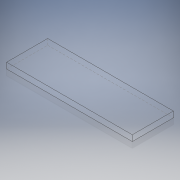
# Autodesk Inventor part: Door Shelf
Saved by Autodesk Inventor 2016 (Build 200138000, 138)
## iProperties
Created: 2017-10-31
Part Number: Door Shelf
Material: Wood (Cherry)
Document SubType Name: Modeling
Designer: mathaetaes
Density: 0.63 g/cm^3
Appearance: Cherry - Natural Low Gloss
Author: mathaetaes
Autodesk Inventor part; units mm, degrees
ref_plane "YZ Plane" through (0, 0, 0) normal (1, 0, 0) x (0, 1, 0)
ref_plane "XZ Plane" through (0, 0, 0) normal (0, 1, 0) x (-1, 0, 0)
ref_plane "XY Plane" through (0, 0, 0) normal (0, 0, 1) x (1, 0, 0)
sketch "Sketch1" plane through (0, 0, 0) normal (0, 1, 0) x (-1, 0, 0)
  line L0 (0, -133.35) -> (-388.9375, -133.35)
  line L1 (-388.9375, -133.35) -> (-388.9375, 0)
  line L2 (-388.9375, 0) -> (0, 0)
  line L3 (0, 0) -> (0, -133.35)
  dimension "d0" = 388.9375
  dimension "d1" = 133.35
  constraints: 8 end point, 2 parallel, 1 coincident, 1 horizontal, 1 perpendicular
  measures "d0" distance of L1.end L2.end
  measures "d1" distance of L0.end L1.end
extrude "Extrusion1" add sketch "Sketch1" along normal blind 19.05
body "Solid1"
